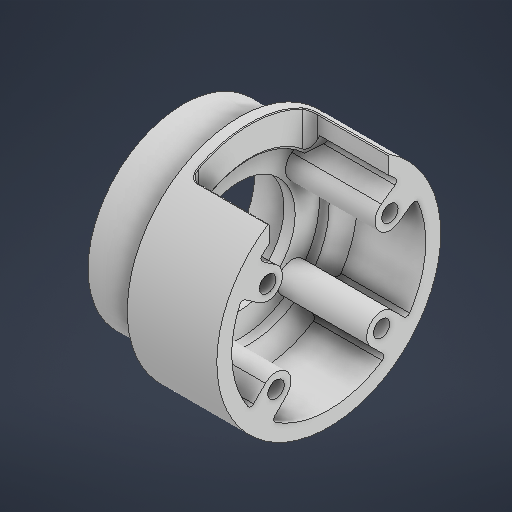
# Autodesk Inventor part: P_Lagerschale
Saved by Autodesk Inventor 2026 (Build 300175000, 175)
## iProperties
Created: 2025-04-25
Part Number: P_Lagerschale
Material: Generisch
Document SubType Name: Modeling
Designer: FAL
Density: 1 g/cm^3
Appearance: Vorgabe
Author: FAL
Autodesk Inventor part; units mm, degrees
ref_plane "YZ Plane" through (0, 0, 0) normal (1, 0, 0) x (0, 1, 0)
ref_plane "XZ Plane" through (0, 0, 0) normal (0, 1, 0) x (-1, 0, 0)
ref_plane "XY Plane" through (0, 0, 0) normal (0, 0, 1) x (1, 0, 0)
sketch "Skizze1" plane through (0, 0, 0) normal (0, 1, 0) x (-1, 0, 0)
  line L0 (0, 0) -> (27.8247, 0)
  line L1 (0, 7.5) -> (0, 10.75)
  line L2 (0, 12.75) -> (7.5, 12.75)
  line L3 (7.5, 12.75) -> (7.5, 9.6)
  line L4 (7.5, 9.6) -> (1.5, 9.6)
  line L5 (1.5, 9.6) -> (1.5, 7.5)
  line L6 (1.5, 7.5) -> (0, 7.5)
  line L7 (0, 7.5) -> (0, 0) construction
  line L8 (0, 10.75) -> (-1.3, 10.75)
  line L9 (-12, 13) -> (-12, 15)
  line L10 (0, 12.75) -> (0, 15)
  line L11 (0, 15) -> (-12, 15)
  line L12 (-12, 13) -> (-2.8, 13)
  line L13 (-2.8, 13) -> (-1.3, 10.75)
  point P0 (4.5, 9.6)
  dimension "d0" = 25.5
  dimension "d1" = 15
  dimension "d2" = 19.2
  dimension "d3" = 6
  dimension "d4" = 1.5
  dimension "d12" = 12
  dimension "d13" = 2
  dimension "d33" = 30
  dimension "d34" = 2
  dimension "d35" = 1.3
  dimension "d36" = 1.5
  constraints: 29 end point, 10 perpendicular, 2 collinear, 2 horizontal, 2 point on line, 1 midpoint, 1 vertical
  measures "d0" diameter of L2 L0
  measures "d1" diameter of L6 L0
  measures "d2" diameter of point (4.5, 9.6) L0
  measures "d3" distance between parallel lines of L3 L5
  measures "d4" distance between parallel lines of L5 L1
  measures "d12" distance between parallel lines of L1 L9
  measures "d13" distance between parallel lines of L8 L2
  measures "d33" diameter of L11 L0
  measures "d34" distance between parallel lines of L11 L12
  measures "d35" distance from line of L1 L8.end
  measures "d36" horizontal distance of L12.end L8.end
revolve "Umdrehung1" add sketch "Skizze1" angle 360 about axis through (0, 0, 0) along (-1, 0, 0)
sketch "Skizze3" plane through (-7.5, 0, 0) normal (-1, 0, 0) x (0, 0, 1)
  circle A0 centre (0, 0) radius 12.75 projected
  line L0 (0, 12.75) -> (0, 9.6) construction
  circle A1 centre (0, 0) radius 9.6 projected
  circle A2 centre (0, 11.175) radius 0.95
  dimension "d6" = 1.9
  constraints: 2 end point, 2 vertical alignment, 1 centre point, 1 midpoint, 1 vertical, 2 other
  measures "d6" diameter of A2
extrude "Extrusion1" cut sketch "Skizze3" against normal blind 4 contours A2
pattern_circular "Runde Anordnung1" count 3 over 360 about axis through (-4.5, 0, 0) along (-1, 0, 0) of "Extrusion1"
sketch "Skizze4" plane through (0, 0, 0) normal (0, 0, 1) x (1, 0, 0)
  line L0 (18.5, -8) -> (1.5, -8)
  line L1 (1.5, -8) -> (1.5, 8)
  line L2 (1.5, 8) -> (18.5, 8)
  line L3 (18.5, 8) -> (18.5, -8)
  line L4 (10, 12.75) -> (10, -12.75) projected
  line L5 (18.5, -8) -> (1.5, 8) construction
  line L6 (1.5, -8) -> (18.5, 8) construction
  line L7 (0, 10.75) -> (0, -10.75) projected
  point P0 (0, 0)
  point P1 (10, 0)
  dimension "d14" = 16
  dimension "d20" = 1.5
  constraints: 12 end point, 3 midpoint, 2 parallel, 1 horizontal, 1 perpendicular
  measures "d14" distance between parallel lines of L2 L0
  measures "d20" distance between parallel lines of L7 L1
extrude "Extrusion2" cut sketch "Skizze4" along normal blind 18
fillet "Rundung1" radius 1 2 edges at (1.5, 8, 10.1555) (1.5, -8, 10.1555)
sketch "Skizze5" plane through (0, 0, 0) normal (1, 0, 0) x (0, 0, -1)
  arc A0 (-4.0975, -9.3387) -> (-7.3741, -7.0444) centre (-5.7358, -8.1915) ccw
  line L0 (-7.3741, -7.0444) -> (-10.1651, -11.0304)
  line L1 (-6.8885, -13.3247) -> (-4.0975, -9.3387)
  line L2 (-5.7358, -8.1915) -> (0, 0) construction
  arc A1 (-10.1651, -11.0304) -> (-6.8885, -13.3247) centre (0, 0) ccw
  line L3 (0, 0) -> (0, -12.75) construction
  circle A2 centre (0, 0) radius 15 projected
  dimension "d21" = 2
  dimension "d22" = 10
  dimension "d32" = 35
  constraints: 8 end point, 4 point on circle, 2 centre point, 2 coincident, 2 parallel, 2 tangent, 1 concentric, 1 vertical
  measures "d21" radius of A0
  measures "d22" distance of L2.end L2.start
  measures "d32" angle of L3 L2
extrude "Extrusion3" add sketch "Skizze5" along normal up to surface (12 mm away) contours L1 A1 L0 A0
sketch "Skizze6" plane through (12, 0, 0) normal (1, 0, 0) x (0, 0.6699732, -0.7423853)
  arc A0 (-9.2986, -4.1877) -> (-10.1939, -0.2892) centre (-9.7462, -2.2385) ccw projected
  circle A1 centre (-9.7462, -2.2385) radius 1.1
  point P0 (0, 0)
  point P1 (6.097, 8.8537)
  point P2 (8.2731, 6.8643)
  dimension "d25" = 2.2
  constraints: 1 centre point, 1 coincident
  measures "d25" diameter of A1
extrude "Extrusion4" cut sketch "Skizze6" against normal blind 6.75
fillet "Rundung4" radius 0.5 2 edges at (7.4, -9.375, 9.006) (7.4, -11.6694, 5.7294)
pattern_circular "Runde Anordnung2" count 2 over 80 about axis through (0.65, 0, 0) along (1, 0, 0) of "Extrusion3", "Extrusion4", "Rundung4"
mirror "Spiegeln1" about plane through (0, 0, 0) normal (0, 1, 0) of "Extrusion3", "Extrusion4", "Runde Anordnung2", "Rundung4"
fillet "Rundung3" radius 0.1 6 edges at (1.8055, 7.7195, 12.8612) (7.25, 8, 12.6886) (1.8055, -7.7195, 12.8612) (7.25, -8, 12.6886) (1.5, 3.6057, 14.5602) (1.5, -3.6057, 14.5602)
ref_plane "Arbeitsebene1" through (0, 0, 0) normal (0, 1, 0) x (-1, 0, 0)
